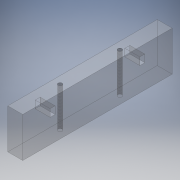
# Autodesk Inventor part: ImagineFrameFront
Saved by Autodesk Inventor 2018 (Build 220112000, 112)
## iProperties
Created: 2020-09-26
Part Number: ImagineFrameFront
Material: Polycarbonate, Clear
Document SubType Name: Modeling
Designer: Lveli
Density: 1.2 g/cm^3
Appearance: Polycarbonate - Clear
Author: Lveli
Autodesk Inventor part; units mm, degrees
ref_plane "YZ Plane" through (0, 0, 0) normal (1, 0, 0) x (0, 1, 0)
ref_plane "XZ Plane" through (0, 0, 0) normal (0, 1, 0) x (-1, 0, 0)
ref_plane "XY Plane" through (0, 0, 0) normal (0, 0, 1) x (1, 0, 0)
sketch "Sketch1" plane through (0, 0, 0) normal (0, 0, 1) x (1, 0, 0)
  line L0 (0, 0) -> (9.525, 0)
  line L1 (9.525, 0) -> (9.525, 25.4)
  line L2 (9.525, 25.4) -> (0, 25.4)
  line L3 (0, 25.4) -> (0, 0)
  dimension "d0" = 9.525
  dimension "d1" = 25.4
  constraints: 8 end point, 2 parallel, 1 horizontal, 1 perpendicular
  measures "d0" distance of L2.end L1.end
  measures "d1" distance of L1.end L0.end
extrude "Extrusion1" add sketch "Sketch1" along normal blind 95.25
sketch "Sketch2" plane through (0, 25.4, 0) normal (0, 1, 0) x (1, 0, 0)
  line L0 (0, 0) -> (0, -95.25) construction
  line L1 (0, -47.625) -> (9.525, -47.625) construction
  line L2 (9.525, 0) -> (9.525, -95.25) construction
  point P0 (4.7625, -19.05)
  point P1 (4.7625, -76.2)
  dimension "d4" = 19.05
  dimension "d5" = 4.7625
  constraints: 2 end point, 2 midpoint, 1 symmetric about line
  measures "d4" vertical distance of L0.start point (4.763, -19.05)
  measures "d5" distance from line of L0 point (4.763, -19.05)
hole "Hole1" at (4.7625, 25.4, 19.05) at (4.7625, 25.4, 76.2) direction (0, -1, 0) diameter 2.6416 end through all thread size "6-32 UNC" class "2B" standard "ANSI Unified Screw Threads"
sketch "Sketch3" plane through (0, 0, 0) normal (-1, 0, 0) x (0, 0, 1)
  line L0 (0, 25.4) -> (0, 0) construction
  line L1 (0, 0) -> (95.25, 0) construction
  line L2 (95.25, 25.4) -> (95.25, 0) construction
  line L3 (0, 25.4) -> (95.25, 25.4) construction
  line L4 (7.9375, 19.8438) -> (11.1125, 19.8438)
  line L5 (11.1125, 19.8438) -> (11.1125, 15.0812)
  line L6 (11.1125, 15.0812) -> (7.9375, 15.0812)
  line L7 (7.9375, 15.0812) -> (7.9375, 19.8438)
  line L8 (7.9375, 19.8438) -> (11.1125, 15.0812) construction
  line L9 (11.1125, 19.8438) -> (7.9375, 15.0812) construction
  line L10 (0, 0) -> (95.25, 0) construction
  line L11 (47.625, 0) -> (47.625, 25.4) construction
  line L12 (87.3125, 19.8438) -> (84.1375, 19.8438)
  line L13 (84.1375, 19.8438) -> (84.1375, 15.0813)
  line L14 (84.1375, 15.0813) -> (87.3125, 15.0813)
  line L15 (87.3125, 15.0813) -> (87.3125, 19.8438)
  line L16 (87.3125, 19.8438) -> (84.1375, 15.0813) construction
  line L17 (84.1375, 19.8438) -> (87.3125, 15.0813) construction
  point P0 (9.525, 17.4625)
  point P1 (85.725, 17.4625)
  dimension "d13" = 3.175
  dimension "d14" = 4.7625
  dimension "d15" = 9.525
  dimension "d16" = 7.9375
  constraints: 26 end point, 6 midpoint, 5 symmetric about line, 2 parallel, 1 horizontal, 1 perpendicular
  measures "d13" distance of L5.end L6.end
  measures "d14" distance of L6.end L4.start
  measures "d15" distance from line of L0 point (9.525, 17.463)
  measures "d16" distance from line of L3 point (9.525, 17.463)
extrude "Extrusion2" cut sketch "Sketch3" against normal through all
body "Solid1"
